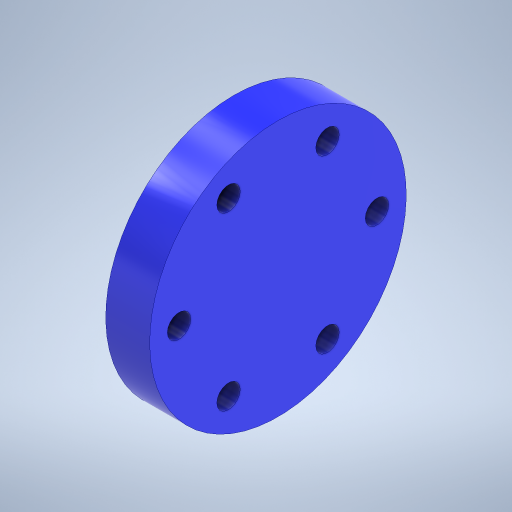
# Autodesk Inventor part: link5_plate1
Saved by Autodesk Inventor 2024 (Build 280153000, 153)
## iProperties
Created: 2024-12-13
Part Number: link5_plate1
Material: ABS プラスチック
Document SubType Name: Modeling
Designer: hirek
Density: 1.06 g/cm^3
Appearance: 青 - 壁塗料 - 光沢
Author: hirek
Autodesk Inventor part; units mm, degrees
ref_plane "YZ Plane" through (0, 0, 0) normal (1, 0, 0) x (0, 1, 0)
ref_plane "XZ Plane" through (0, 0, 0) normal (0, 1, 0) x (-1, 0, 0)
ref_plane "XY Plane" through (0, 0, 0) normal (0, 0, 1) x (1, 0, 0)
sketch "スケッチ1" plane through (0, 0, 0) normal (1, 0, 0) x (0, 1, 0)
  circle A0 centre (0, 0) radius 17.5
  dimension "d0" = 35
  constraints: 1 centre point, 1 coincident
  measures "d0" diameter of A0
extrude "押し出し1" add sketch "スケッチ1" along normal blind 6
sketch "スケッチ2" plane through (6, 0, 0) normal (1, 0, 0) x (0, 0, -1)
  circle A0 centre (0, 0) radius 13.5
  point P0 (13.5, 0)
  point P1 (6.75, 11.6913)
  point P2 (-6.75, 11.6913)
  point P3 (-13.5, 0)
  point P4 (-6.75, -11.6913)
  point P5 (6.75, -11.6913)
  dimension "d3" = 27
  dimension "d6" = 360
  constraints: 1 coincident, 1 horizontal alignment, 9 other
hole "穴1" at (6, 0, -13.5) at (6, 11.6913, -6.75) at (6, 11.6913, 6.75) at (6, 0, 13.5) at (6, -11.6913, 6.75) at (6, -11.6913, -6.75) direction (-1, 0, 0) diameter 3.2 end through all
